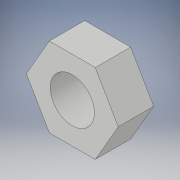
# Autodesk Inventor part: RobotArm Nut
Saved by Autodesk Inventor 2018 (Build 220112000, 112)
## iProperties
Created: 2018-01-20
Part Number: RobotArm Nut
Material: Generic
Document SubType Name: Modeling
Designer: lopez.xavier
Density: 1 g/cm^3
Appearance: Default
Author: lopez.xavier
Autodesk Inventor part; units mm, degrees
ref_plane "YZ Plane" through (0, 0, 0) normal (1, 0, 0) x (0, 1, 0)
ref_plane "XZ Plane" through (0, 0, 0) normal (0, 1, 0) x (-1, 0, 0)
ref_plane "XY Plane" through (0, 0, 0) normal (0, 0, 1) x (1, 0, 0)
sketch "Sketch1" plane through (0, 0, 0) normal (0, 0, 1) x (1, 0, 0)
  line L0 (3.2996, 5.715) -> (6.5991, 0)
  line L1 (6.5991, 0) -> (3.2996, -5.715)
  line L2 (3.2996, -5.715) -> (-3.2996, -5.715)
  line L3 (-3.2996, -5.715) -> (-6.5991, 0)
  line L4 (-6.5991, 0) -> (-3.2996, 5.715)
  line L5 (-3.2996, 5.715) -> (3.2996, 5.715)
  line L6 (0, 0) -> (0.811, 0)
  circle A0 centre (0, 0) radius 3.175
  dimension "d0" = 11.43
  dimension "d1" = 6.35
  constraints: 14 end point, 2 coincident, 1 centre point, 1 horizontal, 1 parallel, 13 other
  measures "d0" distance between parallel lines of L2 L5
  measures "d1" diameter of A0
extrude "Extrusion1" add sketch "Sketch1" along normal blind 5.08
body "Solid1"
